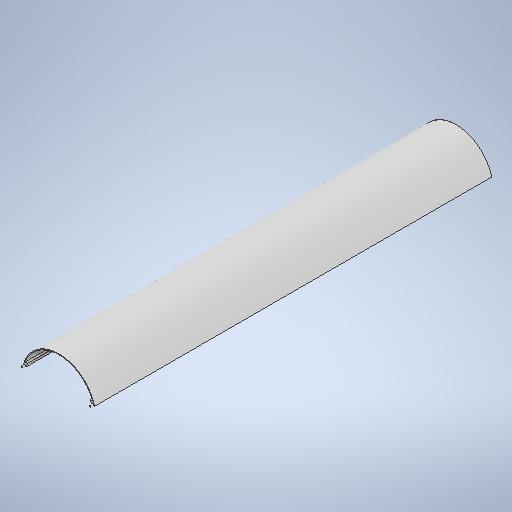
# Autodesk Inventor part: PCB Tray Top
Saved by Autodesk Inventor 2025 (Build 290162000, 162)
## iProperties
Created: 2024-07-12
Part Number: PCB Tray Top
Material: Generic
Document SubType Name: Modeling
Designer: track
Density: 1 g/cm^3
Appearance: Default
Author: track
## iProperties of the stored document PCB Tray Top_3DPrint.ipt
Created: 2024-07-12
Part Number: PCB Tray Top_3DPrint
Material: Generic
Document SubType Name: Modeling
Designer: track
Density: 1 g/cm^3
Appearance: Default
Author: track
Autodesk Inventor part; units mm, degrees
ref_plane "YZ Plane" through (0, 0, 0) normal (1, 0, 0) x (0, 1, 0)
ref_plane "XZ Plane" through (0, 0, 0) normal (0, 1, 0) x (-1, 0, 0)
ref_plane "XY Plane" through (0, 0, 0) normal (0, 0, 1) x (1, 0, 0)
sketch "Sketch1" plane through (0, 0, 0) normal (0, 0, 1) x (1, 0, 0)
  circle A0 centre (0, 0) radius 25.4
  circle A1 centre (0, 0) radius 23.4
  dimension "d0" = 50.8
  dimension "d1" = 2
  constraints: 2 centre point, 1 coincident
  measures "d0" diameter of A0
  measures "d1" radial gap between concentric circles of A0 A1
extrude "Extrusion1" add sketch "Sketch1" against normal blind 274
sketch "Sketch2" plane through (0, 0, 0) normal (0, 0, 1) x (1, 0, 0)
  line L0 (-25.4, 6.35) -> (25.4, 6.35)
  line L1 (25.4, 6.35) -> (25.4, -25.4)
  line L2 (25.4, -25.4) -> (-25.4, -25.4)
  line L3 (-25.4, -25.4) -> (-25.4, 6.35)
  circle A0 centre (0, 0) radius 25.4 projected
  line L4 (0, 25.4) -> (0, -25.4)
  point P0 (-24.5934, 6.35)
  point P1 (24.5934, 6.35)
  dimension "d6" = 25.4
  dimension "d7" = 25.4
  dimension "d8" = 25.4
  dimension "d9" = 19.05
  constraints: 10 end point, 2 parallel, 2 point on circle, 1 horizontal, 1 midpoint, 1 perpendicular, 1 vertical
  measures "d6" distance from line of A0.centre L2
  measures "d7" distance from line of A0.centre L1
  measures "d8" distance from line of A0.centre L3
  measures "d9" distance from line of L4.start L0
extrude "Extrusion2" cut sketch "Sketch2" against normal through all contours L0 L4 A0 | L0 A0 L4 picked at (-1.884, -14.6044) picked at (1.884, -14.6044)
sketch "Sketch3" plane through (0, 0, 0) normal (0, 0, 1) x (1, 0, 0)
  line L0 (22.5219, 6.35) -> (24.5934, 6.35) projected
  line L1 (23.5577, 6.35) -> (23.5577, 9.4971)
  arc A0 (24.5934, 6.35) -> (-24.5934, 6.35) centre (0, 0) ccw projected
  circle A1 centre (23.5577, 6.85) radius 0.5
  line L2 (0, 25.4) -> (0, 6.35) construction
  circle A2 centre (-23.5577, 6.85) radius 0.5
  dimension "d12" = 1
  dimension "d13" = 0.5
  constraints: 4 end point, 2 centre point, 2 point on circle, 2 vertical, 1 midpoint, 1 point on line, 1 symmetric about line, 1 other
  measures "d12" diameter of A1
  measures "d13" distance from line of L0 A1.centre
extrude "Extrusion3" add sketch "Sketch3" along normal blind 2 contours A1 L1 | L1 A1 | A2
sketch "Sketch4" plane through (0, 0, 0) normal (0, 0, 1) x (1, 0, 0)
  arc A0 (23.2589, 8.89) -> (-23.2589, 8.89) centre (0, 0) ccw
  arc A1 (24.5934, 6.35) -> (-24.5934, 6.35) centre (0, 0) ccw projected
  arc A2 (21.6455, 8.89) -> (-21.6455, 8.89) centre (0, 0) ccw
  arc A3 (22.5219, 6.35) -> (-22.5219, 6.35) centre (0, 0) ccw projected
  line L0 (-23.2589, 8.89) -> (-21.6455, 8.89)
  line L1 (23.2589, 8.89) -> (21.6455, 8.89)
  line L2 (22.5219, 6.35) -> (23.5577, 6.35) projected
  dimension "d17" = 0.5
  dimension "d18" = 2.54
  constraints: 6 point on circle, 5 end point, 2 centre point, 2 coincident, 2 concentric, 2 point on line, 1 horizontal
  measures "d17" radial gap between concentric circles of A1 A0
  measures "d18" distance between parallel lines of L2 L1
extrude "Extrusion4" cut sketch "Sketch4" against normal through all
body "Solid1"
